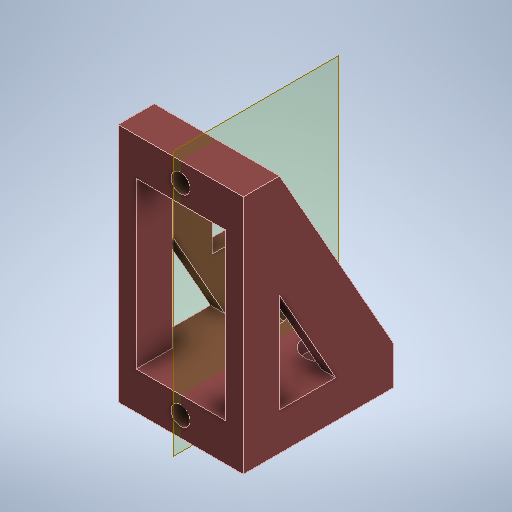
# Autodesk Inventor part: GrabberServoHolder
Saved by Autodesk Inventor 2025.1 (Build 291241000, 241)
## iProperties
Created: 2025-02-23
Part Number: GrabberServoHolder
Material: Generic
Document SubType Name: Modeling
Designer: 13156
Density: 1 g/cm^3
Appearance: Default
Author: 13156
## iProperties of the stored document GrabberServoHolder_3DPrint.ipt
Created: 2025-02-23
Part Number: GrabberServoHolder_3DPrint
Material: Generic
Document SubType Name: Modeling
Designer: jerem
Density: 1 g/cm^3
Appearance: Default
Author: jerem
Autodesk Inventor part; units mm, degrees
ref_plane "YZ Plane" through (0, 0, 0) normal (1, 0, 0) x (0, 1, 0)
ref_plane "XZ Plane" through (0, 0, 0) normal (0, 1, 0) x (-1, 0, 0)
ref_plane "XY Plane" through (0, 0, 0) normal (0, 0, 1) x (1, 0, 0)
sketch "Sketch1" plane through (0, 0, 0) normal (0, 0, 1) x (1, 0, 0)
  line L0 (-8.65, 16.6) -> (8.65, 16.6)
  line L1 (8.65, 16.6) -> (8.65, -16.6)
  line L2 (8.65, -16.6) -> (-8.65, -16.6)
  line L3 (-8.65, -16.6) -> (-8.65, 16.6)
  line L4 (0, 0) -> (0, 2.5695) construction
  line L5 (0, 0) -> (15.5803, 0) construction
  line L6 (-6.15, 11.4) -> (6.15, 11.4)
  line L7 (6.15, 11.4) -> (6.15, -11.4)
  line L8 (6.15, -11.4) -> (-6.15, -11.4)
  line L9 (-6.15, -11.4) -> (-6.15, 11.4)
  circle A0 centre (-0.0401, 13.9) radius 1.3
  circle A1 centre (-0.0401, -13.9) radius 1.3
  line L10 (-13.4961, 0) -> (20.4264, 0) projected
  line L11 (8.65, -16.6) -> (-8.65, -16.6)
  line L12 (-8.65, -16.6) -> (-8.65, -11.4)
  line L13 (-8.65, -11.4) -> (8.65, -11.4)
  line L14 (8.65, -11.4) -> (8.65, -16.6)
  point P0 (0, 16.6)
  dimension "d0" = 2.6
  dimension "d1" = 27.8
  dimension "d2" = 0.0401
  dimension "d4" = 12.3
  dimension "d5" = 2.5
  dimension "d6" = 2.5
  dimension "d7" = 22.8
  dimension "d11" = 2.7
  dimension "d12" = 2.7
  dimension "d14" = 2.5
  constraints: 28 end point, 6 parallel, 4 horizontal, 3 perpendicular, 2 centre point, 1 collinear, 1 equal radius, 1 midpoint, 1 point on line, 1 vertical, 3 other
  measures "d0" diameter of A0
  measures "d1" distance of A1.centre A0.centre
  measures "d2" distance from line of L4 A0.centre
  measures "d4" distance of L7.end L8.end
  measures "d5" distance from line of L6 A0.centre
  measures "d6" distance from line of L8 A1.centre
  measures "d7" distance between parallel lines of L8 L6
  measures "d11" vertical distance of point (0, 16.6) A0.centre
  measures "d12" distance from line of L2 A1.centre
  measures "d14" distance between parallel lines of L7 L1
extrude "Extrusion1" add sketch "Sketch1" along normal blind 5 contours L0 L1 L10 L7 L6 L9 L3 | L10 L9 L13 L3 | L1 L13 L7 L10 | L13 L8 L1 L2 L3
extrude "Extrusion2" add sketch "Sketch1" against normal blind 15.8 contours L13 L8 L1 L2 L3
sketch "Sketch2" plane through (-6.15, -11.4, 5) normal (0, 1, 0) x (1, 0, 0)
  circle A0 centre (10.3, 15.485) radius 1.05
  circle A1 centre (2, 15.485) radius 1.05
  line L0 (-2.5, 20.8) -> (14.8, 20.8) projected
  line L1 (-2.5, 5) -> (-2.5, 20.8) projected
  point P0 (6.15, 5)
  dimension "d19" = 2.1
  dimension "d20" = 0
  dimension "d21" = 5.315
  dimension "d22" = 8.3
  dimension "d23" = 4.5
  constraints: 2 centre point, 1 equal radius
  measures "d19" diameter of A0
  measures "d20" vertical distance of A0.centre A1.centre
  measures "d21" distance from line of L0 A1.centre
  measures "d22" distance of A1.centre A0.centre
  measures "d23" distance from line of L1 A1.centre
extrude "Extrusion3" cut sketch "Sketch2" against normal blind 10
sketch "Sketch3" plane through (-6.15, -11.4, 5) normal (0, 1, 0) x (1, 0, 0)
  circle A0 centre (10.3, 15.485) radius 1.05 projected
  circle A1 centre (10.3, 15.485) radius 2.5
  circle A2 centre (2, 15.485) radius 1.05 projected
  circle A3 centre (2, 15.485) radius 2.5
  point P0 (6.15, 5)
  dimension "d26" = 5
  constraints: 2 centre point, 2 coincident, 1 equal radius
  measures "d26" diameter of A1
extrude "Extrusion4" cut sketch "Sketch3" against normal blind 2
sketch "Sketch4" plane through (8.65, -11.4, 0) normal (1, 0, 0) x (0, 0, -1)
  line L0 (0, 0) -> (15.8, 0) projected
  line L1 (0, 0) -> (0, 28) projected
  line L2 (15.8, 0) -> (0, 28)
  line L3 (0, 28) -> (0, 13.7562)
  line L4 (0, 13.7562) -> (7.7624, 0)
  line L5 (7.7624, 0) -> (15.8, 0)
  line L6 (0, 28) -> (-5, 28) projected
  line L7 (0, 13.7562) -> (0, 28)
  line L8 (6, 17.3671) -> (11.2857, 17.3671)
  line L9 (11.2857, 17.3671) -> (11.2857, 8)
  line L10 (11.2857, 8) -> (6, 8)
  line L11 (6, 8) -> (6, 17.3671)
  point P0 (0, 11.4)
  dimension "d29" = 7
  dimension "d33" = 8
  dimension "d34" = 6
  constraints: 18 end point, 4 point on line, 3 parallel, 2 perpendicular, 1 horizontal
  measures "d29" distance between parallel lines of L4 L2
  measures "d33" distance between parallel lines of L0 L10
  measures "d34" horizontal distance of L3.end L8.start
ref_plane "Work Plane1" through (0, -11.4, 0) normal (-1, 0, 0) x (0, 0, 1)
extrude "Extrusion5" add sketch "Sketch4" against normal blind 2 contours L4 L1 L2 L11 L10 L0 | L10 L11 L2
mirror "Mirror1" about plane through (0, -11.4, 0) normal (-1, 0, 0) of "Extrusion5"
extrude "Extrusion6" cut sketch "Sketch4" against normal blind 12.2875 from surface at -8.65 contours L10 L11 L2
body "Solid1"
